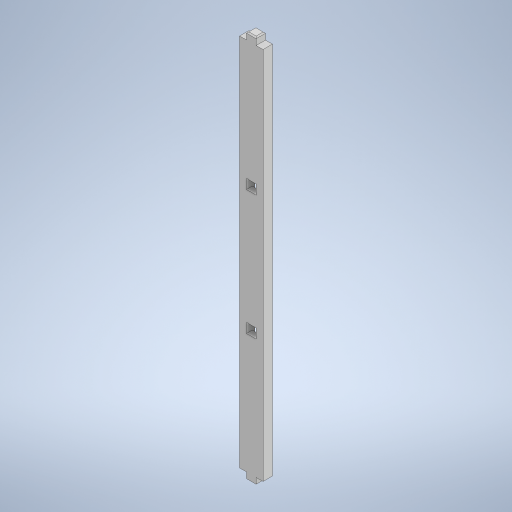
# Autodesk Inventor part: BareCalibrationClipSide
Saved by Autodesk Inventor 2024 (Build 280153000, 153)
## iProperties
Created: 2024-03-12
Part Number: BareCalibrationClipSide
Material: Generic
Document SubType Name: Modeling
Designer: jevan
Density: 1 g/cm^3
Appearance: Default
Author: jevan
Autodesk Inventor part; units mm, degrees
ref_plane "YZ Plane" through (0, 0, 0) normal (1, 0, 0) x (0, 1, 0)
ref_plane "XZ Plane" through (0, 0, 0) normal (0, 1, 0) x (-1, 0, 0)
ref_plane "XY Plane" through (0, 0, 0) normal (0, 0, 1) x (1, 0, 0)
sketch "Sketch1" plane through (0, 0, 0) normal (0, 0, 1) x (1, 0, 0)
  line L0 (5, 82.875) -> (-5, 82.875)
  line L1 (-5, 82.875) -> (-5, -82.875)
  line L2 (-5, -82.875) -> (5, -82.875)
  line L3 (5, -82.875) -> (5, 82.875)
  line L4 (-2.05, 24.575) -> (2.05, 24.575)
  line L5 (2.05, 24.575) -> (2.05, 28.675)
  line L6 (2.05, 28.675) -> (-2.05, 28.675)
  line L7 (-2.05, 28.675) -> (-2.05, 24.575)
  line L8 (-2.05, -24.575) -> (2.05, -24.575)
  line L9 (2.05, -24.575) -> (2.05, -28.675)
  line L10 (2.05, -28.675) -> (-2.05, -28.675)
  line L11 (-2.05, -28.675) -> (-2.05, -24.575)
  line L12 (0, -28.675) -> (0, 28.675)
  line L13 (-5, 0) -> (0, 0)
  line L14 (-2.05, 82.875) -> (-2.05, 79.875)
  line L15 (-2.05, 79.875) -> (-5, 79.875)
  line L16 (2.05, 82.875) -> (2.05, 79.875)
  line L17 (2.05, 79.875) -> (5, 79.875)
  line L18 (-2.05, -82.875) -> (-2.05, -79.875)
  line L19 (-2.05, -79.875) -> (-5, -79.875)
  line L20 (2.05, -82.875) -> (2.05, -79.875)
  line L21 (2.05, -79.875) -> (5, -79.875)
  dimension "d0" = 10
  dimension "d1" = 165.75
  dimension "d4" = 4.1
  dimension "d5" = 4.1
  dimension "d6" = 49.15
  dimension "d7" = 4.1
  dimension "d8" = 4.1
  dimension "d9" = 5
  dimension "d10" = 3
  dimension "d11" = 3
  constraints: 44 end point, 12 point on line, 9 perpendicular, 6 parallel, 5 midpoint, 4 collinear, 4 horizontal, 1 vertical
  measures "d0" distance of L0.start L0.end
  measures "d1" distance of L2.end L0.start
  measures "d4" distance of L6.end L5.end
  measures "d5" distance between parallel lines of L4 L6
  measures "d6" distance between parallel lines of L8 L4
  measures "d7" distance between parallel lines of L10 L8
  measures "d8" distance between parallel lines of L9 L11
  measures "d9" distance between parallel lines of L3 L12
  measures "d10" distance of L14.start L14.end
  measures "d11" distance of L18.start L18.end
extrude "Extrusion1" add sketch "Sketch1" along normal blind 4 contours L16 L17 L3 L21 L20 L2 L18 L19 L1 L15 L14 L0
chamfer "Chamfer1" distance 0.5 angle 45 12 edges at (0, 82.875, 4) (-2.05, 82.875, 2) (0, 82.875, 0) (2.05, 82.875, 2) (2.05, -82.875, 2) (0, -82.875, 4) (-2.05, -82.875, 2) (0, -82.875, 0) (2.05, 26.625, 0) (-2.05, 26.625, 0) (2.05, -26.625, 0) (-2.05, -26.625, 0)
chamfer "Chamfer2" distance 1.5 angle 45 12 edges at (2.3, 28.675, 0) (0, 28.675, 0) (-2.3, 28.675, 0) (2.3, 24.575, 0) (0, 24.575, 0) (-2.3, 24.575, 0) (2.3, -24.575, 0) (0, -24.575, 0) (-2.3, -24.575, 0) (2.3, -28.675, 0) (0, -28.675, 0) (-2.3, -28.675, 0)
equation "\"d5\" = d4"
equation "\"d7\" = d4"
equation "\"d8\" = d4"
equation "\"d9\" = 0.5 * d0"
body "Solid1"
